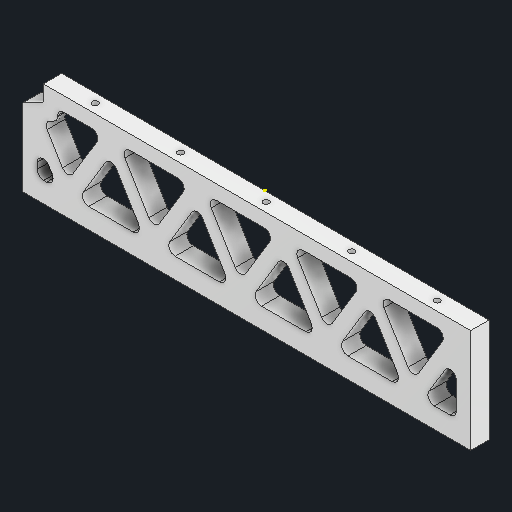
# Autodesk Inventor part: LeftTruss
Saved by Autodesk Inventor 2026.2 (Build 302298000, 298)
## iProperties
Created: 2026-04-01
Part Number: LeftTruss
Material: ABS Plastic
Document SubType Name: Modeling
Designer: gaoet
Density: 1.06 g/cm^3
Appearance: Smooth - White
Author: gaoet
Autodesk Inventor part; units mm, degrees
ref_plane "YZ Plane" through (0, 0, 0) normal (1, 0, 0) x (0, 1, 0)
ref_plane "XZ Plane" through (0, 0, 0) normal (0, 1, 0) x (-1, 0, 0)
ref_plane "XY Plane" through (0, 0, 0) normal (0, 0, 1) x (1, 0, 0)
sketch "Sketch1" plane through (0, 0, 0) normal (0, 0, 1) x (1, 0, 0)
  line L0 (-110, -25.5) -> (110, -25.5)
  line L1 (110, -25.5) -> (110, 25.5)
  line L2 (110, 25.5) -> (-110, 25.5)
  line L3 (-110, 25.5) -> (-110, -25.5)
  line L4 (-110, -25.5) -> (110, 25.5) construction
  line L5 (110, -25.5) -> (-110, 25.5) construction
  line L6 (-110, 17.5) -> (-100, 17.5)
  line L7 (-100, 17.5) -> (-100, 25.5)
  point P0 (0, 0)
  dimension "d0" = 220
  dimension "d1" = 51
  dimension "d2" = 10
  dimension "d3" = 8
  constraints: 16 end point, 2 horizontal, 2 midpoint, 2 parallel, 2 perpendicular, 2 point on line
  measures "d0" distance of L2.end L1.end
  measures "d1" distance of L0.end L1.end
  measures "d2" distance of L6.start L6.end
  measures "d3" distance of L6.end L7.end
extrude "Extrusion1" add sketch "Sketch1" along normal blind 9 contours L3 L6 L7 L2 L1 L0
chamfer "Chamfer1" distance 10 distance2 5 1 edges at (-110, 17.5, 4.5) measured on face at (-109.5, 17.5, 4.5)
sketch "Sketch2" plane through (-110, -25.5, 0) normal (0, -1, 0) x (1, 0, 0)
  line L0 (0, 0) -> (0, 9) projected
  line L1 (0, 0) -> (220, 0) projected
  point P0 (110, 0)
  point P1 (22, 4.5)
  point P2 (42, 4.5)
  point P3 (62, 4.5)
  point P4 (82, 4.5)
  point P5 (102, 4.5)
  point P6 (122, 4.5)
  point P7 (142, 4.5)
  point P8 (162, 4.5)
  point P9 (182, 4.5)
  point P10 (202, 4.5)
  dimension "d9" = 22
  dimension "d10" = 4.5
  dimension "d13" = 20
  constraints: 1 horizontal, 9 other
  measures "d9" distance from line of L0 point (22, 4.5)
  measures "d10" distance from line of L1 point (22, 4.5)
  measures "d13" distance of point (22, 4.5) point (42, 4.5)
hole "Hole1" at (-88, -25.5, 4.5) at (-68, -25.5, 4.5) at (-48, -25.5, 4.5) at (-28, -25.5, 4.5) at (-8, -25.5, 4.5) at (12, -25.5, 4.5) at (32, -25.5, 4.5) at (52, -25.5, 4.5) at (72, -25.5, 4.5) at (92, -25.5, 4.5) direction (0, 1, 0) diameter 3 depth 9
sketch "Sketch3" plane through (0, 0, 9) normal (0, 0, 1) x (1, 0, 0)
  line L0 (-89.5, -16.5) -> (-86.5, -16.5) projected
  line L1 (-110, 12.5) -> (-110, -25.5) projected
  line L2 (-110, -16.5) -> (110, -16.5)
  line L3 (110, -25.5) -> (110, 25.5) projected
  line L4 (-110, 12.5) -> (-100, 17.5) projected
  line L5 (-110, 12.5) -> (-110, -25.5) projected
  line L6 (-110, -25.5) -> (110, -25.5) projected
  line L7 (110, -25.5) -> (110, 25.5) projected
  line L8 (110, 25.5) -> (-100, 25.5) projected
  line L9 (-100, 25.5) -> (-100, 17.5) projected
  line L10 (-93, 18.5) -> (103, 18.5)
  line L11 (103, 18.5) -> (103, -18.5)
  line L12 (103, -18.5) -> (-103, -18.5)
  line L13 (-103, -18.5) -> (-103, 8.1738)
  line L14 (-103, 8.1738) -> (-93, 13.1738)
  line L15 (-93, 13.1738) -> (-93, 18.5)
  line L16 (103, 18.5) -> (81.7738, -16.5) construction
  line L17 (60.5475, 18.5) -> (81.7738, -16.5) construction
  line L18 (39.3213, -16.5) -> (60.5475, 18.5) construction
  line L19 (18.095, 18.5) -> (39.3213, -16.5) construction
  line L20 (-3.1312, -16.5) -> (18.095, 18.5) construction
  line L21 (-3.1312, -16.5) -> (-24.3575, 18.5) construction
  line L22 (-45.5837, -16.5) -> (-24.3575, 18.5) construction
  line L23 (-89.5, -16.5) -> (-86.5, -16.5) projected
  line L24 (-28.4508, 18.5) -> (-49.6771, -16.5)
  line L25 (-20.2641, 18.5) -> (-41.4904, -16.5)
  line L26 (-28.4508, 18.5) -> (-7.2246, -16.5)
  line L27 (-20.2641, 18.5) -> (0.9621, -16.5)
  line L28 (14.0016, 18.5) -> (-7.2246, -16.5)
  line L29 (0.9621, -16.5) -> (22.1884, 18.5)
  line L30 (14.0016, 18.5) -> (35.2279, -16.5)
  line L31 (22.1884, 18.5) -> (43.4146, -16.5)
  line L32 (35.2279, -16.5) -> (56.4541, 18.5)
  line L33 (64.6409, 18.5) -> (85.8671, -16.5)
  line L34 (103, 11.7505) -> (85.8671, -16.5)
  line L35 (56.4541, 18.5) -> (77.6804, -16.5)
  line L36 (64.6409, 18.5) -> (43.4146, -16.5)
  line L37 (98.9066, 18.5) -> (77.6804, -16.5)
  line L38 (-45.5837, -16.5) -> (-66.81, 18.5) construction
  line L39 (-66.81, 18.5) -> (-88.0362, -16.5) construction
  line L40 (-103, 8.1738) -> (-88.0362, -16.5) construction
  line L41 (-88.0362, -16.5) -> (-109.2625, 18.5) construction
  line L42 (-62.7166, 18.5) -> (-40.9509, -17.3896)
  line L43 (-70.9033, 18.5) -> (-49.6771, -16.5)
  line L44 (-92.1296, -16.5) -> (-70.9033, 18.5)
  line L45 (-62.7166, 18.5) -> (-83.9429, -16.5)
  line L46 (-99.8591, 9.7442) -> (-83.9429, -16.5)
  line L47 (-103, 1.4242) -> (-92.1296, -16.5)
  point P0 (0, 0)
  point P1 (49.9344, 1)
  point P2 (103, -16.5)
  point P3 (18.095, 11.7505)
  point P4 (81.7738, -9.7505)
  point P5 (60.5475, 11.7505)
  point P6 (39.3213, -9.7505)
  point P7 (-3.1312, -9.7505)
  point P8 (-24.3575, 11.7505)
  point P9 (-103, -16.5)
  point P10 (-95.5181, -4.1631)
  point P11 (-45.5837, -9.7505)
  point P12 (-66.81, 11.7505)
  point P13 (-88.0362, -9.7505)
  dimension "d25" = 7
  dimension "d32" = 3.5
  dimension "d33" = 3.5
  dimension "d34" = 3.5
  dimension "d35" = 3.5
  dimension "d36" = 3.5
  dimension "d37" = 3.5
  dimension "d38" = 3.5
  dimension "d39" = 3.5
  dimension "d40" = 3.5
  dimension "d41" = 3.5
  dimension "d42" = 3.5
  dimension "d43" = 3.5
  dimension "d44" = 3.5
  dimension "d46" = 3.5
  dimension "d67" = 58.765
  dimension "d68" = 3.5
  dimension "d69" = 3.5
  dimension "d70" = 3.5
  dimension "d71" = 3.5
  dimension "d72" = 3.5
  dimension "d73" = 3.5
  constraints: 72 end point, 20 parallel, 9 equal length, 5 point on line, 2 midpoint, 1 collinear, 1 horizontal, 1 horizontal alignment, 56 other
  measures "d32" distance between parallel lines of L22 L24
  measures "d33" distance between parallel lines of L25 L22
  measures "d34" distance between parallel lines of L26 L21
  measures "d35" distance between parallel lines of L21 L27
  measures "d36" distance between parallel lines of L20 L28
  measures "d37" distance between parallel lines of L20 L29
  measures "d38" distance between parallel lines of L19 L30
  measures "d39" distance between parallel lines of L19 L31
  measures "d40" distance from line of point (49.934, 1) L32
  measures "d41" distance between parallel lines of L36 L18
  measures "d42" distance between parallel lines of L17 L35
  measures "d43" distance between parallel lines of L17 L33
  measures "d44" distance between parallel lines of L16 L34
  measures "d46" distance between parallel lines of L16 L37
  measures "d67" angle to the sketch x axis of L27
  measures "d68" distance between parallel lines of L38 L42
  measures "d69" distance between parallel lines of L43 L38
  measures "d70" distance between parallel lines of L39 L45
  measures "d71" distance between parallel lines of L39 L44
  measures "d72" distance between parallel lines of L40 L46
  measures "d73" distance from line of L47 point (-95.518, -4.163)
extrude "Extrusion2" cut sketch "Sketch3" against normal through all contours L2 L13 L47 | L45 L43 L2 | L46 L14 L15 L10 L44 | L25 L26 L2 | L42 L10 L24 | L2 L34 L11 | L29 L30 L2 | L27 L10 L28 | L2 L36 L35 | L33 L10 L37 | L31 L10 L32
fillet "Fillet1" radius 3 33 edges at (-93, 18.5, 4.5) (-93, 13.1738, 4.5) (-103, -16.5, 4.5) (-24.3575, 11.7505, 4.5) (-28.4508, 18.5, 4.5) (-41.4904, -16.5, 4.5) (-3.1312, -9.7505, 4.5) (-20.2641, 18.5, 4.5) (14.0016, 18.5, 4.5) (0.9621, -16.5, 4.5) (18.095, 11.7505, 4.5) (39.3213, -9.7505, 4.5) (22.1884, 18.5, 4.5) (103, -16.5, 4.5) (85.8671, -16.5, 4.5) (103, 11.7505, 4.5) (98.9066, 18.5, 4.5) (64.6409, 18.5, 4.5) (56.4541, 18.5, 4.5) (60.5475, 11.7505, 4.5) (43.4146, -16.5, 4.5) (77.6804, -16.5, 4.5) (81.7738, -9.7505, 4.5) (-99.8591, 9.7442, 4.5) (-70.9033, 18.5, 4.5) (-62.7166, 18.5, 4.5) (-49.6771, -16.5, 4.5) (-66.81, 11.7505, 4.5) (-83.9429, -16.5, 4.5) (-88.0362, -9.7505, 4.5) (-103, 1.4242, 4.5) (-92.1296, -16.5, 4.5) (-45.5837, -9.7505, 4.5)
sketch "Sketch4" plane through (-100, 25.5, 0) normal (0, 1, 0) x (1, 0, 0)
  point P0 (100, 0)
sketch "Sketch5" plane through (-100, 25.5, 0) normal (0, 1, 0) x (1, 0, 0)
  line L0 (210, 0) -> (210, -9) projected
  line L1 (0, 0) -> (0, -9) projected
  line L2 (210, 0) -> (0, 0) projected
  point P0 (100, 0)
  point P1 (21, -4.5)
  point P2 (63, -4.5)
  point P3 (105, -4.5)
  point P4 (147, -4.5)
  point P5 (189, -4.5)
  dimension "d50" = 210
  dimension "d51" = 21
  dimension "d52" = 42
  dimension "d53" = 42
  dimension "d54" = 42
  dimension "d55" = 4.5
  dimension "d78" = 42
  constraints: 4 horizontal alignment
  measures "d50" distance between parallel lines of L0 L1
  measures "d51" distance from line of L1 point (21, -4.5)
  measures "d52" distance of point (63, -4.5) point (21, -4.5)
  measures "d53" distance of point (105, -4.5) point (63, -4.5)
  measures "d54" distance of point (147, -4.5) point (105, -4.5)
  measures "d55" distance from line of L2 point (21, -4.5)
  measures "d78" distance of point (189, -4.5) point (147, -4.5)
hole "Hole2" at (-37, 25.5, 4.5) at (-79, 25.5, 4.5) at (5, 25.5, 4.5) at (47, 25.5, 4.5) at (89, 25.5, 4.5) direction (0, -1, 0) diameter 3 depth 10
sketch "Sketch8" plane through (0, 0, 9) normal (0, 0, 1) x (1, 0, 0)
  arc A0 (-73.6662, 13.9443) -> (-76.2313, 18.5) centre (-76.2313, 15.5) ccw projected
  line L0 (-73.6662, 13.9443) -> (-85.4711, -5.5208) projected
  arc A1 (-90.6014, -5.5208) -> (-85.4711, -5.5208) centre (-88.0362, -3.9651) ccw projected
  line L1 (-90.6014, -5.5208) -> (-98.1711, 6.961) projected
  arc A2 (-96.9477, 11.1999) -> (-98.1711, 6.961) centre (-95.606, 8.5167) ccw projected
  line L2 (-96.9477, 11.1999) -> (-94.6584, 12.3446) projected
  arc A3 (-94.6584, 12.3446) -> (-93, 15.0279) centre (-96, 15.0279) ccw projected
  line L3 (79.2086, -5.5208) -> (67.4037, 13.9443) projected
  line L4 (96.1438, 13.9443) -> (84.3389, -5.5208) projected
  arc A4 (79.2086, -5.5208) -> (84.3389, -5.5208) centre (81.7738, -3.9651) ccw projected
  line L5 (-7.2246, -16.5) -> (-36.1624, -16.5) projected
  arc A5 (-38.7275, -11.9443) -> (-36.1624, -16.5) centre (-36.1624, -13.5) ccw projected
  line L6 (-38.7275, -11.9443) -> (-26.9226, 7.5208) projected
  arc A6 (-21.7924, 7.5208) -> (-26.9226, 7.5208) centre (-24.3575, 5.9651) ccw projected
  line L7 (-21.7924, 7.5208) -> (-7.2246, -16.5) projected
  line L8 (-31.2137, 13.9443) -> (-43.0186, -5.5208) projected
  arc A7 (-48.1489, -5.5208) -> (-43.0186, -5.5208) centre (-45.5837, -3.9651) ccw projected
  line L9 (-48.1489, -5.5208) -> (-59.9538, 13.9443) projected
  arc A8 (-57.3887, 18.5) -> (-59.9538, 13.9443) centre (-57.3887, 15.5) ccw projected
  line L10 (63.1126, 7.5208) -> (74.9176, -11.9443) projected
  arc A9 (72.3524, -16.5) -> (74.9176, -11.9443) centre (72.3524, -13.5) ccw projected
  line L11 (72.3524, -16.5) -> (48.7426, -16.5) projected
  arc A10 (46.1775, -11.9443) -> (48.7426, -16.5) centre (48.7426, -13.5) ccw projected
  line L12 (46.1775, -11.9443) -> (57.9824, 7.5208) projected
  arc A11 (63.1126, 7.5208) -> (57.9824, 7.5208) centre (60.5475, 5.9651) ccw projected
  line L13 (35.2279, -16.5) -> (6.2901, -16.5) projected
  arc A12 (3.725, -11.9443) -> (6.2901, -16.5) centre (6.2901, -13.5) ccw projected
  line L14 (3.725, -11.9443) -> (15.5299, 7.5208) projected
  arc A13 (20.6601, 7.5208) -> (15.5299, 7.5208) centre (18.095, 5.9651) ccw projected
  line L15 (20.6601, 7.5208) -> (35.2279, -16.5) projected
  line L16 (-5.6964, -5.5208) -> (-17.5013, 13.9443) projected
  line L17 (11.2388, 13.9443) -> (-0.5661, -5.5208) projected
  arc A14 (-5.6964, -5.5208) -> (-0.5661, -5.5208) centre (-3.1312, -3.9651) ccw projected
  line L18 (-64.2449, 7.5208) -> (-52.4399, -11.9443) projected
  arc A15 (-55.0051, -16.5) -> (-52.4399, -11.9443) centre (-55.0051, -13.5) ccw projected
  line L19 (-55.0051, -16.5) -> (-78.6149, -16.5) projected
  arc A16 (-81.18, -11.9443) -> (-78.6149, -16.5) centre (-78.6149, -13.5) ccw projected
  line L20 (-81.18, -11.9443) -> (-69.3751, 7.5208) projected
  arc A17 (-64.2449, 7.5208) -> (-69.3751, 7.5208) centre (-66.81, 5.9651) ccw projected
  line L21 (-97.4576, -16.5) -> (-100, -16.5) projected
  arc A18 (-103, -13.5) -> (-100, -16.5) centre (-100, -13.5) ccw projected
  line L22 (-103, -13.5) -> (-103, -9.3078) projected
  arc A19 (-97.4349, -7.7521) -> (-103, -9.3078) centre (-100, -9.3078) ccw projected
  line L23 (-97.4349, -7.7521) -> (-94.8924, -11.9443) projected
  arc A20 (-97.4576, -16.5) -> (-94.8924, -11.9443) centre (-97.4576, -13.5) ccw projected
  line L24 (36.7561, -5.5208) -> (24.9512, 13.9443) projected
  line L25 (53.6913, 13.9443) -> (41.8864, -5.5208) projected
  arc A21 (36.7561, -5.5208) -> (41.8864, -5.5208) centre (39.3213, -3.9651) ccw projected
  line L26 (103, 1.0184) -> (103, -13.5) projected
  arc A22 (100, -16.5) -> (103, -13.5) centre (100, -13.5) ccw projected
  line L27 (100, -16.5) -> (91.1951, -16.5) projected
  arc A23 (88.6299, -11.9443) -> (91.1951, -16.5) centre (91.1951, -13.5) ccw projected
  line L28 (88.6299, -11.9443) -> (97.4349, 2.5741) projected
  arc A24 (103, 1.0184) -> (97.4349, 2.5741) centre (100, 1.0184) ccw projected
  line L29 (-110, 12.5) -> (-100, 17.5) projected
  line L30 (-110, 12.5) -> (-110, -25.5) projected
  line L31 (-110, -25.5) -> (110, -25.5) projected
  line L32 (110, -25.5) -> (110, 25.5) projected
  line L33 (110, 25.5) -> (-100, 25.5) projected
  line L34 (-100, 25.5) -> (-100, 17.5) projected
  line L35 (110, -15.5) -> (-110, -15.5)
  line L36 (-93, 15.0279) -> (-93, 15.5) projected
  arc A25 (-90, 18.5) -> (-93, 15.5) centre (-90, 15.5) ccw projected
  line L37 (-90, 18.5) -> (-76.2313, 18.5) projected
  arc A26 (69.9688, 18.5) -> (67.4037, 13.9443) centre (69.9688, 15.5) ccw projected
  line L38 (69.9688, 18.5) -> (93.5787, 18.5) projected
  arc A27 (96.1438, 13.9443) -> (93.5787, 18.5) centre (93.5787, 15.5) ccw projected
  line L39 (-57.3887, 18.5) -> (-33.7788, 18.5) projected
  arc A28 (-31.2137, 13.9443) -> (-33.7788, 18.5) centre (-33.7788, 15.5) ccw projected
  arc A29 (-14.9362, 18.5) -> (-17.5013, 13.9443) centre (-14.9362, 15.5) ccw projected
  line L40 (-14.9362, 18.5) -> (8.6737, 18.5) projected
  arc A30 (11.2388, 13.9443) -> (8.6737, 18.5) centre (8.6737, 15.5) ccw projected
  arc A31 (27.5163, 18.5) -> (24.9512, 13.9443) centre (27.5163, 15.5) ccw projected
  line L41 (27.5163, 18.5) -> (51.1262, 18.5) projected
  arc A32 (53.6913, 13.9443) -> (51.1262, 18.5) centre (51.1262, 15.5) ccw projected
  point P0 (0, 0)
  point P1 (102.2361, -15.5)
  point P2 (88.959, -15.5)
  point P3 (74.5885, -15.5)
  point P4 (46.5065, -15.5)
  point P5 (34.6214, -15.5)
  point P6 (4.054, -15.5)
  point P7 (-95.2215, -15.5)
  point P8 (-102.2361, -15.5)
  point P9 (-52.769, -15.5)
  point P10 (-80.851, -15.5)
  point P11 (-7.8311, -15.5)
  point P12 (-38.3985, -15.5)
  dimension "d74" = 10
  constraints: 2 end point, 2 point on line, 1 horizontal
  measures "d74" distance between parallel lines of L31 L35
extrude "Extrusion4" add sketch "Sketch8" against normal up to surface (9 mm away) contours L5 A5 L35 L7 | L35 L15 L13 A12 | A15 L19 A16 L35 | L35 A9 L11 A10 | A20 L21 A18 L35 | L35 A22 L27 A23
fillet "Fillet3" radius 3.175 12 edges at (-102.2361, -15.5, 4.5) (-95.2215, -15.5, 4.5) (-80.851, -15.5, 4.5) (-52.769, -15.5, 4.5) (-38.3985, -15.5, 4.5) (-7.8311, -15.5, 4.5) (4.054, -15.5, 4.5) (34.6214, -15.5, 4.5) (46.5065, -15.5, 4.5) (74.5885, -15.5, 4.5) (88.959, -15.5, 4.5) (102.2361, -15.5, 4.5)
equation "\"d32\" = 0.5 * d25"
equation "\"d33\" = 0.5 * d25"
equation "\"d34\" = 0.5 * d25"
equation "\"d35\" = 0.5 * d25"
equation "\"d36\" = 0.5 * d25"
equation "\"d37\" = 0.5 * d25"
equation "\"d38\" = 0.5 * d25"
equation "\"d39\" = 0.5 * d25"
equation "\"d40\" = 0.5 * d25"
equation "\"d41\" = 0.5 * d25"
equation "\"d42\" = 0.5 * d25"
equation "\"d43\" = 0.5 * d25"
equation "\"d44\" = 0.5 * d25"
equation "\"d46\" = 0.5 * d25"
equation "\"d52\" = 2 * d51"
equation "\"d53\" = d52"
equation "\"d54\" = d53"
body "Solid1"
